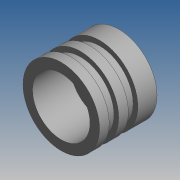
# Autodesk Inventor part: P003-Corps_piston
Saved by Autodesk Inventor 2021.4 (Build 254397000, 397)
## iProperties
Created: 2022-03-18
Part Number: P003-Corps_piston
Material: Générique
Document SubType Name: Modeling
Designer: Maintenant Prêt
Density: 1 g/cm^3
Appearance: Par défaut
Author: Maintenant Prêt
Autodesk Inventor part; units mm, degrees
ref_plane "YZ Plane" through (0, 0, 0) normal (1, 0, 0) x (0, 1, 0)
ref_plane "XZ Plane" through (0, 0, 0) normal (0, 1, 0) x (-1, 0, 0)
ref_plane "XY Plane" through (0, 0, 0) normal (0, 0, 1) x (1, 0, 0)
sketch "Sketch5" plane through (0, 0, 0) normal (0, 0, 1) x (1, 0, 0)
  line L0 (-24, 0) -> (4, 0) construction
  line L1 (0, -6) -> (0, 36) construction
  line L2 (-15, 0) -> (-15, 20)
  line L3 (-15, 20) -> (0, 20)
  line L4 (0, 30) -> (-20, 30)
  line L5 (-20, 30) -> (-20, 20)
  line L6 (-20, 20) -> (-17.5, 20)
  line L7 (-17.5, 20) -> (-17.5, 15)
  line L8 (-17.5, 15) -> (-20, 15)
  line L9 (-20, 15) -> (-20, 10)
  line L10 (-20, 10) -> (-17.5, 10)
  line L11 (-17.5, 10) -> (-17.5, 5)
  line L12 (-17.5, 5) -> (-20, 5)
  line L13 (-20, 5) -> (-20, 0)
  line L14 (-20, 0) -> (-17.5, 0)
  line L15 (-17.5, 0) -> (-17.5, 5)
  line L16 (-17.5, 5) -> (-20, 5)
  line L17 (-20, 5) -> (-20, 0)
  line L18 (0, 30) -> (0, 20)
  line L19 (-20, 0) -> (-15, 0)
  point P0 (0, 0)
  dimension "d13" = 10
  dimension "d14" = 10
  dimension "d15" = 5
  dimension "d16" = 5
  dimension "d17" = 5
  dimension "d18" = 5
  dimension "d19" = 5
  dimension "d20" = 5
  dimension "d21" = 5
  dimension "d22" = 15
  dimension "d23" = 2.5
  constraints: 36 end point, 14 point on line, 9 perpendicular, 2 collinear, 1 horizontal, 1 vertical
  measures "d13" distance of L4.end L5.end
  measures "d14" distance from line of L4 L2.end
  measures "d15" distance between parallel lines of L10 L8
  measures "d16" distance of L10.end L11.end
  measures "d17" distance of L12.end L13.end
  measures "d18" distance of L6.end L7.end
  measures "d19" distance of L16.end L17.end
  measures "d20" distance of L14.end L15.end
  measures "d21" distance between parallel lines of L2 L13
  measures "d22" distance between parallel lines of L1 L2
  measures "d23" distance between parallel lines of L2 L11
revolve "Revolution1" add sketch "Sketch5" angle 360 about axis through (0, -10, 0) along (0, 1, 0)
body "Solid3"
